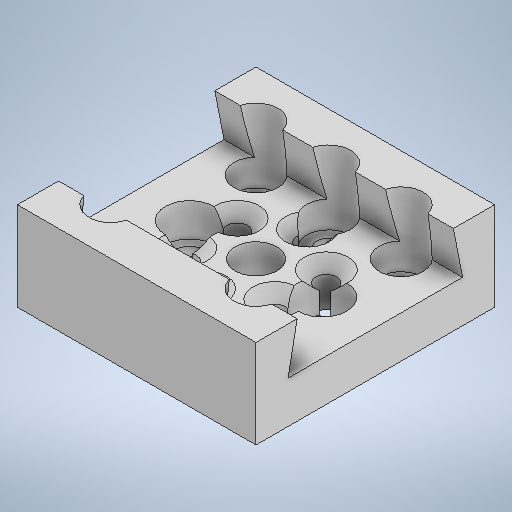
# Autodesk Inventor part: Tube dovetail bracket
Saved by Autodesk Inventor 2025 (Build 290162000, 162)
## iProperties
Created: 2025-08-12
Part Number: Tube dovetail bracket
Material: Generic
Document SubType Name: Modeling
Designer: yshis
Density: 1 g/cm^3
Appearance: Default
Author: yshis
Autodesk Inventor part; units mm, degrees
ref_plane "YZ Plane" through (0, 0, 0) normal (1, 0, 0) x (0, 1, 0)
ref_plane "XZ Plane" through (0, 0, 0) normal (0, 1, 0) x (-1, 0, 0)
ref_plane "XY Plane" through (0, 0, 0) normal (0, 0, 1) x (1, 0, 0)
sketch "Sketch1" plane through (0, 0, 0) normal (0, 1, 0) x (-1, 0, 0)
  line L0 (0, 0) -> (62.6, 0)
  line L1 (62.6, 0) -> (62.6, -62.6)
  line L2 (62.6, -62.6) -> (0, -62.6)
  line L3 (0, -62.6) -> (0, 0)
  circle A0 centre (31.3, -31.3) radius 2.5
  circle A1 centre (12.25, -12.25) radius 3.1
  circle A2 centre (31.3, -12.25) radius 3.1
  circle A3 centre (50.35, -12.25) radius 3.1
  circle A4 centre (12.25, -50.35) radius 3.1
  circle A5 centre (31.3, -50.35) radius 3.1
  circle A6 centre (50.35, -50.35) radius 3.1
  point P0 (31.3, -62.6)
  dimension "d0" = 62.6
  dimension "d1" = 62.6
  dimension "d2" = 5
  dimension "d3" = 31.3
  dimension "d4" = 31.3
  dimension "d5" = 19.05
  dimension "d6" = 19.05
  dimension "d7" = 6.2
  dimension "d10" = 19.05
  dimension "d13" = 38.1
  constraints: 8 end point, 7 centre point, 2 horizontal, 2 parallel, 1 midpoint, 1 perpendicular, 1 vertical, 10 other
  measures "d0" distance of L1.end L2.end
  measures "d1" distance of L0.end L1.end
  measures "d2" diameter of A0
  measures "d3" distance of point (31.3, -62.6) A0.centre
  measures "d4" distance from line of A0.centre L3
  measures "d5" horizontal distance of A1.centre A0.centre
  measures "d6" horizontal distance of A1.centre A0.centre
  measures "d7" diameter of A1
  measures "d10" distance of A1.centre A2.centre
  measures "d13" distance of A1.centre A4.centre
extrude "Extrusion1" add sketch "Sketch1" along normal blind 11 contours L0 L1 L2 L3 | A0 | A2
sketch "Sketch3" plane through (0, 11, 0) normal (0, 1, 0) x (1, 0, 0)
  circle A0 centre (-31.3, 31.3) radius 2.5
  line L0 (-62.6, 0) -> (0, 0) projected
  line L1 (0, 0) -> (0, 62.6) projected
  dimension "d47" = 5
  dimension "d48" = 31.3
  dimension "d49" = 31.3
  constraints: 1 centre point
  measures "d47" diameter of A0
  measures "d48" distance from line of A0.centre L0
  measures "d49" distance from line of A0.centre L1
extrude "Extrusion3" cut sketch "Sketch3" against normal blind 11
sketch "Sketch4" plane through (0, 11, 0) normal (0, 1, 0) x (1, 0, 0)
  circle A0 centre (-31.3, 31.3) radius 2.5 projected
  circle A1 centre (-31.3, 31.3) radius 5.5
  point P0 (0, 0)
  dimension "d52" = 11
  constraints: 1 centre point, 1 coincident
  measures "d52" diameter of A1
sketch "Sketch5" plane through (0, 11, 0) normal (0, 1, 0) x (1, 0, 0)
  circle A0 centre (-12.25, 12.25) radius 3.1 projected
  circle A1 centre (-12.25, 12.25) radius 5.75
  circle A2 centre (-50.35, 12.25) radius 3.1 projected
  circle A3 centre (-50.35, 12.25) radius 5.75
  circle A4 centre (-50.35, 50.35) radius 3.1 projected
  circle A5 centre (-50.35, 50.35) radius 5.75
  circle A6 centre (-31.3, 50.35) radius 3.1 projected
  circle A7 centre (-31.3, 50.35) radius 5.75
  circle A8 centre (-12.25, 50.35) radius 3.1 projected
  circle A9 centre (-12.25, 50.35) radius 5.75
  point P0 (0, 0)
  dimension "d53" = 11.5
  dimension "d54" = 11.5
  dimension "d55" = 11.5
  dimension "d56" = 11.5
  dimension "d57" = 11.5
  constraints: 5 centre point, 5 coincident
  measures "d53" diameter of A1
  measures "d54" diameter of A3
  measures "d55" diameter of A5
  measures "d56" diameter of A7
  measures "d57" diameter of A9
extrude "Extrusion4" cut sketch "Sketch5" against normal blind 7 contours A0 | A1 | A2 | A3 | A4 | A5 | A7 | A8 | A9
extrude "Extrusion5" cut sketch "Sketch4" against normal blind 8
sketch "Sketch7" plane through (0, 11, 0) normal (0, 1, 0) x (1, 0, 0)
  circle A0 centre (-31.3, 31.3) radius 2.5 projected
  circle A1 centre (-31.3, 31.3) radius 1
  circle A2 centre (-48.7, 31.3) radius 4.05
  circle A3 centre (-13.9, 31.3) radius 4.05
  point P0 (0, 0)
  dimension "d63" = 2
  dimension "d64" = 8.1
  dimension "d65" = 17.4
  dimension "d66" = 8.1
  dimension "d67" = 17.4
  constraints: 3 centre point, 1 coincident
  measures "d63" diameter of A1
  measures "d64" diameter of A2
  measures "d65" distance of A1.centre A2.centre
  measures "d66" diameter of A3
  measures "d67" distance of A1.centre A3.centre
extrude "Extrusion6" cut sketch "Sketch7" against normal blind 11 contours A2 | A3
sketch "Sketch8" plane through (0, 11, 0) normal (0, 1, 0) x (1, 0, 0)
  circle A0 centre (-48.7, 31.3) radius 4.05 projected
  circle A1 centre (-48.7, 31.3) radius 6.4
  circle A2 centre (-13.9, 31.3) radius 4.05 projected
  circle A3 centre (-13.9, 31.3) radius 6.4
  point P0 (0, 0)
  point P1 (-44.65, 31.3)
  point P2 (-44.65, 31.3)
  point P3 (-9.85, 31.3)
  point P4 (-9.85, 31.3)
  point P5 (-44.65, 31.3)
  point P6 (-44.65, 31.3)
  dimension "d70" = 12.8
  dimension "d71" = 12.8
  constraints: 2 centre point, 2 coincident
  measures "d70" diameter of A1
  measures "d71" diameter of A3
extrude "Extrusion7" cut sketch "Sketch8" against normal blind 8.7 contours A0 | A1 | A2 | A3
sketch "Sketch9" plane through (0, 11, 0) normal (0, 1, 0) x (1, 0, 0)
  circle A0 centre (-31.3, 31.3) radius 1
  line L0 (-62.6, 0) -> (0, 0) projected
  line L1 (0, 0) -> (0, 62.6) projected
  circle A1 centre (-31.3, 44.8) radius 2.75
  circle A2 centre (-42.9913, 38.05) radius 2.75
  circle A3 centre (-42.9913, 24.55) radius 2.75
  circle A4 centre (-31.3, 17.8) radius 2.75
  circle A5 centre (-19.6087, 24.55) radius 2.75
  circle A6 centre (-19.6087, 38.05) radius 2.75
  dimension "d86" = 2
  dimension "d87" = 31.3
  dimension "d88" = 31.3
  dimension "d89" = 5.5
  dimension "d90" = 13.5
  dimension "d93" = 360
  constraints: 7 centre point, 13 other
  measures "d86" diameter of A0
  measures "d87" distance from line of L0 A0.centre
  measures "d88" distance from line of A0.centre L1
  measures "d89" diameter of A1
  measures "d90" distance of A0.centre A1.centre
extrude "Extrusion8" cut sketch "Sketch9" against normal blind 11 contours A1 | A2 | A3 | A4 | A5 | A6
chamfer "Chamfer3" distance 3 angle 45 10 edges at (-43.6279, 11, -40.7253) (-41.3597, 11, -35.8363) (-41.3597, 11, -26.7637) (-43.6279, 11, -21.8747) (-34.05, 11, -17.8) (-16.9334, 11, -25.1866) (-21.8223, 11, -22.9184) (-21.8223, 11, -39.6816) (-16.9334, 11, -37.4134) (-31.3, 11, -42.05)
sketch "Sketch10" plane through (0, 0, 0) normal (1, 0, 0) x (0, 0, -1)
  line L0 (62.6, 11) -> (0, 11) projected
  line L1 (62.6, 11) -> (62.6, 23.3)
  line L2 (62.6, 23.3) -> (51.8, 23.3)
  line L3 (51.8, 23.3) -> (54.2, 11)
  line L4 (54.2, 11) -> (62.6, 11)
  line L5 (0, 11) -> (0, 23.3)
  line L6 (0, 23.3) -> (10.8, 23.3)
  line L7 (10.8, 23.3) -> (8.4, 11)
  point P0 (0, 0)
  dimension "d67" = 17.4
  dimension "d100" = 12.3
  dimension "d101" = 10.8
  dimension "d102" = 8.4
  dimension "d103" = 12.3
  dimension "d104" = 10.8
  dimension "d105" = 8.4
  constraints: 14 end point, 2 perpendicular, 2 point on line, 2 vertical, 1 collinear
  measures "d100" distance of L0.start L1.end
  measures "d101" distance of L1.end L2.end
  measures "d102" distance of L0.start L3.end
  measures "d103" distance of L0.end L5.end
  measures "d104" distance of L5.end L6.end
  measures "d105" distance of L0.end L7.end
extrude "Extrusion9" add sketch "Sketch10" against normal blind 62.6
sketch "Sketch11" plane through (0, 11, 0) normal (0, 1, 0) x (1, 0, 0)
  circle A0 centre (-50.35, 12.25) radius 5.75
  circle A1 centre (-50.35, 50.35) radius 3.1 projected
  circle A2 centre (-50.35, 50.35) radius 5.75
  arc A3 (-30.3772, 47.3905) -> (-32.2228, 47.3905) centre (-31.3, 50.35) ccw projected
  circle A4 centre (-31.3, 50.35) radius 5.75
  circle A5 centre (-12.25, 50.35) radius 5.75
  circle A6 centre (-12.25, 12.25) radius 3.1 projected
  circle A7 centre (-12.25, 12.25) radius 5.75
  point P0 (0, 0)
  constraints: 5 centre point, 5 coincident
extrude "Extrusion10" cut sketch "Sketch11" along normal blind 62.6 contours A0 | A1 | A2 | A4 | A5 | A6 | A7
equation "\"d3\" = 0.5 * d1"
equation "\"d4\" = 0.5 * d0"
equation "\"d48\" = 0.5 * d0"
equation "\"d49\" = 0.5 * d1"
equation "\"d66\" = d64"
equation "\"d67\" = d65"
equation "\"d87\" = 0.5 * d1"
equation "\"d88\" = 0.5 * d0"
equation "\"d106\" = d1"
equation "\"d108\" = d1"
body "Solid1"
